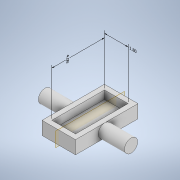
# Autodesk Inventor part: connectorToTubeBrackets
Saved by Autodesk Inventor 2021 (Build 250183000, 183)
## iProperties
Created: 2020-07-21
Part Number: connectorToTubeBrackets
Material: Generic
Document SubType Name: Modeling
Designer: robst
Density: 1 g/cm^3
Appearance: Default
Author: robst
Autodesk Inventor part; units mm, degrees
ref_plane "XZ Plane" through (0, 0, 0) normal (0, 1, 0) x (-1, 0, 0)
ref_plane "XY Plane" through (0, 0, 0) normal (0, 0, 1) x (1, 0, 0)
sketch "Sketch1" plane through (0, 0, 0) normal (0, 1, 0) x (-1, 0, 0)
  line L0 (32.385, 60.325) -> (-32.385, 60.325)
  line L1 (-32.385, 60.325) -> (-32.385, -60.325)
  line L2 (-32.385, -60.325) -> (32.385, -60.325)
  line L3 (32.385, -60.325) -> (32.385, 60.325)
  line L4 (32.385, 60.325) -> (-32.385, -60.325) construction
  line L5 (-32.385, 60.325) -> (32.385, -60.325) construction
  point P0 (0, 0)
  dimension "d0" = 64.77
  dimension "d1" = 120.65
  constraints: 12 end point, 2 midpoint, 2 parallel, 1 horizontal, 1 perpendicular
  measures "d0" distance of L1.end L2.end
  measures "d1" distance of L2.end L0.start
extrude "Extrusion1" add sketch "Sketch1" against normal blind 9.525
sketch "Sketch2" plane through (0, 0, 0) normal (0, 1, 0) x (1, 0, 0)
  line L0 (32.385, -60.325) -> (32.385, 60.325)
  line L1 (32.385, 60.325) -> (-32.385, 60.325)
  line L2 (-32.385, 60.325) -> (-32.385, -60.325)
  line L3 (-32.385, -60.325) -> (32.385, -60.325)
  line L4 (32.385, -60.325) -> (-32.385, 60.325) construction
  line L5 (32.385, 60.325) -> (-32.385, -60.325) construction
  line L6 (22.86, -50.8) -> (22.86, 50.8)
  line L7 (22.86, 50.8) -> (-22.86, 50.8)
  line L8 (-22.86, 50.8) -> (-22.86, -50.8)
  line L9 (-22.86, -50.8) -> (22.86, -50.8)
  line L10 (22.86, -50.8) -> (-22.86, 50.8) construction
  line L11 (22.86, 50.8) -> (-22.86, -50.8) construction
  line L12 (32.385, 60.325) -> (-32.385, 60.325) projected
  line L13 (-32.385, 60.325) -> (-32.385, -60.325) projected
  point P0 (0, 0)
  dimension "wallThickness" = 9.525
  dimension "d5" = 9.525
  constraints: 24 end point, 4 midpoint, 4 parallel, 2 collinear, 2 perpendicular, 1 vertical
  measures "wallThickness" distance between parallel lines of L7 L1
  measures "d5" distance between parallel lines of L2 L8
extrude "Extrusion2" add sketch "Sketch2" along normal blind 15.875
sketch "Sketch3" plane through (32.385, -9.525, 60.325) normal (1, 0, 0) x (0, 0, -1)
  circle A0 centre (56.4652, 12.7) radius 12.7
  line L0 (0, 25.4) -> (120.65, 25.4) projected
  point P0 (60.325, 9.525)
  dimension "d14" = 25.4
  dimension "d15" = 12.7
  constraints: 1 centre point
  measures "d14" diameter of A0
  measures "d15" distance from line of A0.centre L0
extrude "Extrusion3" add sketch "Sketch3" along normal blind 50.8
mirror "Mirror1" about plane through (0, 0, 0) normal (1, 0, 0) of "Extrusion3"
equation "\"d0\" = innerWidth + 2 * wallThickness"
equation "\"d1\" = innerLength + 2 * wallThickness"
equation "\"d2\" = wallThickness"
equation "\"d5\" = wallThickness"
equation "\"innerWidth\" = 45.72"
equation "\"innerLength\" = 101.6"
body "Solid1"
